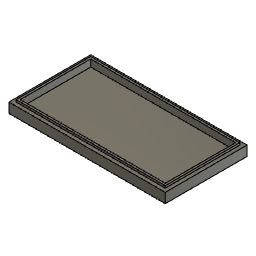
USB Case Cover v1 (Autodesk Fusion 360 design; units mm, degrees)
Autodesk Fusion 360 part; units mm, degrees
sketch "Sketch1" plane through (0, 0, 0) normal (0, 1, 0) x (1, 0, 0)
  line L0 (0, 0) -> (95.5, 0)
  line L1 (95.5, 0) -> (95.5, 50)
  line L2 (95.5, 50) -> (0, 50)
  line L3 (0, 50) -> (0, 0)
  dimension "d1" = 95.5
  dimension "d2" = 50
  constraint horizontal L0
  constraint vertical L1
  constraint horizontal L2
  constraint vertical L3
  constraint coincident L0.start L3.end
  measures "d1" distance of L0.start L0.end
  measures "d2" distance of L0.start L2.end
extrude "Extrude1" add sketch "Sketch1" along normal blind 6
sketch "Sketch3" plane through (0, 6, 0) normal (0, 1, 0) x (-1, 0, 0)
  line L0 (0, -50) -> (0, 0)
  line L1 (0, 0) -> (-95.5, 0)
  line L2 (-95.5, 0) -> (-95.5, -50)
  line L3 (-95.5, -50) -> (0, -50)
  line L4 (-2.2, -2.2) -> (-93.3, -2.2)
  line L5 (-93.3, -2.2) -> (-93.3, -47.8)
  line L6 (-93.3, -47.8) -> (-2.2, -47.8)
  line L7 (-2.2, -47.8) -> (-2.2, -2.2)
  dimension "d7" = 91.1
  dimension "d8" = 45.6
  constraint horizontal L4
  constraint vertical L5
  constraint horizontal L6
  constraint vertical L7
  measures "d7" distance of L4.start L4.end
  measures "d8" distance of L4.start L6.end
extrude "Extrude2" cut sketch "Sketch3" against normal blind 3 contours L4 L5 L6 L7
sketch "Sketch4" plane through (0, 3, 0) normal (0, 1, 0) x (-1, 0, 0)
  line L0 (-2.2, -47.8) -> (-2.2, -2.2)
  line L1 (-2.2, -2.2) -> (-93.3, -2.2)
  line L2 (-93.3, -2.2) -> (-93.3, -47.8)
  line L3 (-93.3, -47.8) -> (-2.2, -47.8)
  line L4 (-3.5, -3.5) -> (-92, -3.5)
  line L5 (-92, -3.5) -> (-92, -46.5)
  line L6 (-92, -46.5) -> (-3.5, -46.5)
  line L7 (-3.5, -46.5) -> (-3.5, -3.5)
  dimension "d11" = 88.5
  dimension "d12" = 43
  constraint horizontal L4
  constraint vertical L5
  constraint horizontal L6
  constraint vertical L7
  measures "d11" distance of L4.start L4.end
  measures "d12" distance of L4.start L6.end
extrude "Extrude3" add sketch "Sketch4" along normal blind 4.3
